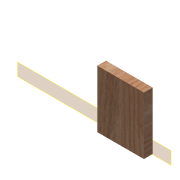
# Autodesk Inventor part: ControllerPlatform
Saved by Autodesk Inventor 2015 (Build 190159000, 159)
## iProperties
Created: 2014-08-03
Part Number: ControllerPlatform
Material: Wood (Birch)
Document SubType Name: Modeling
Designer: david
Density: 0.55 g/cm^3
Appearance: Birch - Natural Polished
Author: david
Autodesk Inventor part; units mm, degrees
ref_plane "YZ Plane" through (0, 0, 0) normal (1, 0, 0) x (0, 1, 0)
ref_plane "XZ Plane" through (0, 0, 0) normal (0, 1, 0) x (-1, 0, 0)
ref_plane "XY Plane" through (0, 0, 0) normal (0, 0, 1) x (1, 0, 0)
ref_plane "Work Plane1" through (0, 0, 0) normal (0, 0, 1) x (1, 0, 0)
sketch "Sketch1" plane through (0, 0, 0) normal (0, 0, 1) x (1, 0, 0)
  line L0 (127, -12.7) -> (25.4, -12.7)
  line L1 (25.4, -12.7) -> (25.4, 112.7506)
  line L2 (25.4, 112.7506) -> (127, 112.7506)
  line L3 (127, 112.7506) -> (127, -12.7)
  line L4 (152.4, -12.7) -> (-152.4, -12.7) projected
  circle A0 centre (133.35, 0) radius 3.175 projected
  circle A1 centre (-146.05, 0) radius 3.175 projected
  circle A2 centre (-133.35, 0) radius 3.175 projected
  circle A3 centre (146.05, 0) radius 3.175 projected
  line L5 (152.4, 12.7) -> (152.4, -12.7) projected
  line L6 (-152.4, 12.7) -> (152.4, 12.7) projected
  line L7 (-152.4, -12.7) -> (-152.4, 12.7) projected
  line L8 (152.4, -12.7) -> (-152.4, -12.7) projected
  circle A4 centre (133.35, 100.0506) radius 3.175 projected
  circle A5 centre (-146.05, 100.0506) radius 3.175 projected
  circle A6 centre (-133.35, 100.0506) radius 3.175 projected
  circle A7 centre (146.05, 100.0506) radius 3.175 projected
  line L9 (152.4, 112.7506) -> (152.4, 87.3506) projected
  line L10 (-152.4, 112.7506) -> (152.4, 112.7506) projected
  line L11 (-152.4, 87.3506) -> (-152.4, 112.7506) projected
  line L12 (152.4, 87.3506) -> (-152.4, 87.3506) projected
  line L13 (127, 12.6746) -> (127, -61.8239) projected
  point P0 (0, 0)
  dimension "d0" = 101.6
  constraints: 8 end point, 3 point on line, 2 parallel, 1 horizontal, 1 perpendicular
  measures "d0" distance of L0.start L0.end
extrude "Extrusion1" add sketch "Sketch1" along normal blind 19.05 contours L0 L1 L6 L3 | L1 L12 L3 L6 | L1 L2 L3 L12
body "Solid1"
